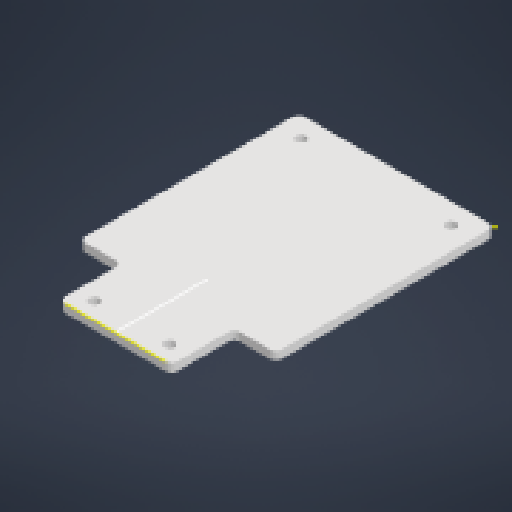
# Autodesk Inventor part: 1.5_base_2
Saved by Autodesk Inventor 2025 (Build 290162010, 162A)
## iProperties
Created: 2024-05-22
Part Number: 1.5_base_2
Material: Generic
Document SubType Name: Modeling
Designer: Garfieldcmix
Density: 1 g/cm^3
Appearance: Default
Author: Garfieldcmix
Autodesk Inventor part; units mm, degrees
ref_plane "YZ Plane" through (0, 0, 0) normal (1, 0, 0) x (0, 1, 0)
ref_plane "XZ Plane" through (0, 0, 0) normal (0, 1, 0) x (-1, 0, 0)
ref_plane "XY Plane" through (0, 0, 0) normal (0, 0, 1) x (1, 0, 0)
derived "Car_Plan.ipt"
sketch "Car_Sketch" plane through (0, 0, 0) normal (0, 1, 0) x (-1, 0, 0)
  line L0 (0, 0) -> (94, 0)
  line L1 (0, 0) -> (0, 105)
  line L2 (94, 0) -> (94, 105)
  line L3 (0, 105) -> (20, 105)
  line L4 (20, 105) -> (20, 190)
  line L5 (20, 190) -> (74, 190)
  line L6 (74, 190) -> (74, 105)
  line L7 (74, 105) -> (94, 105)
  line L8 (-5, 68) -> (-5, 0)
  line L9 (-5, 0) -> (-32, 0)
  line L10 (-32, 0) -> (-32, 68)
  line L11 (-32, 68) -> (-5, 68)
  line L12 (47, 190) -> (47, 0) construction
  line L13 (126, 68) -> (99, 68)
  line L14 (99, 68) -> (99, 0)
  line L15 (126, 0) -> (126, 68)
  line L16 (99, 0) -> (126, 0)
  line L17 (-5, 34) -> (99, 34) construction
  line L18 (0, 95) -> (94, 95) construction
  line L19 (-5, 190) -> (-32, 190)
  line L20 (-32, 122) -> (-5, 122)
  line L21 (-32, 190) -> (-32, 122)
  line L22 (-5, 122) -> (-5, 190)
  line L23 (-5, 156) -> (99, 156) construction
  line L24 (126, 122) -> (99, 122)
  line L25 (126, 190) -> (126, 122)
  line L26 (99, 190) -> (126, 190)
  line L27 (99, 122) -> (99, 190)
  line L28 (0, 156) -> (47, 34) construction
  line L29 (94, 156) -> (47, 34) construction
  line L30 (0, 156) -> (-174.2341, 34) construction
  line L31 (-5, 34) -> (-174.2341, 34) construction
  line L32 (8.9873, 132.6713) -> (47, 141.55) construction
  line L33 (85.0127, 132.6713) -> (47, 141.55) construction
sketch "Base" plane through (0, 0, 0) normal (0, 1, 0) x (-1, 0, 0)
  line L0 (0, 0) -> (0, 105) projected
  line L1 (0, 105) -> (20, 105) projected
  line L2 (20, 105) -> (20, 190) projected
  line L3 (74, 190) -> (74, 105) projected
  line L4 (74, 105) -> (94, 105) projected
  line L5 (94, 0) -> (94, 105) projected
  line L6 (0, 0) -> (94, 0) projected
  line L7 (74, 135) -> (20, 135)
  circle A0 centre (29, 127) radius 2.4
  circle A1 centre (65, 127) radius 2.4
  circle A2 centre (11.1, 10) radius 2.4
  circle A3 centre (82.9, 10) radius 2.4
  dimension "d76" = 30
  dimension "d77" = 4.8
  dimension "d78" = 4.8
  dimension "d79" = 9
  dimension "d80" = 22
  dimension "d81" = 22
  dimension "d82" = 9
  dimension "d83" = 4.8
  dimension "d84" = 4.8
  dimension "d85" = 10
  dimension "d86" = 11.1
  dimension "d87" = 10
  dimension "d88" = 11.1
  constraints: 4 centre point, 2 end point, 2 point on line, 1 perpendicular
  measures "d76" distance between parallel lines of L1 L7
  measures "d77" diameter of A0
  measures "d78" diameter of A1
  measures "d79" distance from line of L2 A0.centre
  measures "d80" distance from line of L1 A0.centre
  measures "d81" distance from line of A1.centre L4
  measures "d82" distance from line of L3 A1.centre
  measures "d83" diameter of A2
  measures "d84" diameter of A3
  measures "d85" distance from line of L6 A2.centre
  measures "d86" distance from line of L0 A2.centre
  measures "d87" distance from line of L6 A3.centre
  measures "d88" distance from line of L5 A3.centre
extrude "Extrusion1" add sketch "Base" along normal blind 4
fillet "Fillet2" radius 3 8 edges at (-20, 2, 105) (0, 2, 105) (0, 2, 0) (-94, 2, 0) (-94, 2, 105) (-74, 2, 105) (-74, 2, 135) (-20, 2, 135)
sketch "Sketch19" plane through (0, 4, 0) normal (0, 1, 0) x (1, 0, 0)
  line L0 (0, -102) -> (0, -3) projected
  line L1 (-17, -105) -> (-3, -105) projected
  line L2 (-94, -3) -> (-94, -102) projected
  line L3 (-91, -105) -> (-77, -105) projected
  line L4 (0, -100.2906) -> (-4.5, -100.2906)
  line L5 (-4.5, -100.2906) -> (-89.5, -100.2906)
  line L6 (-89.5, -100.2906) -> (-89.5, -44.2906)
  line L7 (-89.5, -44.2906) -> (-4.5, -44.2906)
  line L8 (-4.5, -44.2906) -> (-4.5, -100.2906)
  line L9 (-4.5, -100.2906) -> (-8, -100.2906)
  line L10 (-4.5, -96.7906) -> (-4.5, -100.2906)
  circle A0 centre (-28, -96.7906) radius 1.35
  line L11 (-28, -96.7906) -> (-24.5, -96.7906)
  line L12 (-24.5, -96.7906) -> (-24.5, -100.2906)
  line L13 (-24.5, -100.2906) -> (-28, -100.2906)
  line L14 (-28, -100.2906) -> (-28, -96.7906)
  line L15 (-24.5, -100.2906) -> (-89.5, -100.2906)
  line L16 (-89.5, -100.2906) -> (-89.5, -44.2906)
  line L17 (-89.5, -44.2906) -> (-24.5, -44.2906)
  line L18 (-24.5, -44.2906) -> (-24.5, -100.2906)
  line L19 (-57, -100.2906) -> (-57, -87.065)
  line L20 (-24.5, -72.2906) -> (-39.3063, -72.2906)
  circle A1 centre (-86, -96.7906) radius 1.35
  circle A2 centre (-28, -47.7906) radius 1.35
  circle A3 centre (-86, -47.7906) radius 1.35
  point P0 (0, 0)
  dimension "d196" = 4.5
  dimension "d197" = 85
  dimension "d198" = 56
  dimension "d199" = 4.7095
  dimension "d202" = 2.7
  dimension "d203" = 3.5
  dimension "d204" = 23.5
  dimension "d205" = 3.5
  constraints: 34 end point, 6 horizontal, 6 parallel, 4 centre point, 3 perpendicular, 3 symmetric about line, 2 midpoint, 2 point on line, 1 vertical, 3 other
  measures "d196" distance of L4.start L4.end
  measures "d197" distance of L6.end L7.end
  measures "d198" distance of L5.end L6.end
  measures "d199" distance between parallel lines of L1 L4
  measures "d202" diameter of A0
  measures "d203" distance from line of L5 L11.start
  measures "d204" distance from line of L8 L11.start
  measures "d205" distance of L12.end L13.end
extrude "Extrusion12" cut sketch "Sketch19" against normal through all contours L14 L11 A0 | A0 L11 L14 | A1 | A2 | A3
sketch "Sketch20" plane through (0, 4, 0) normal (0, 1, 0) x (1, 0, 0)
  line L0 (0, -102) -> (0, -3) projected
  line L1 (0, -4.0657) -> (-25.4, -4.0657)
  line L2 (-3, 0) -> (-91, 0) projected
  line L3 (-25.4, -4.0657) -> (-68.58, -4.0657)
  line L4 (-68.58, -4.0657) -> (-68.58, -39.6257)
  line L5 (-68.58, -39.6257) -> (-25.4, -39.6257)
  line L6 (-25.4, -39.6257) -> (-25.4, -4.0657)
  line L7 (-25.4, -39.6257) -> (-27.94, -39.6257)
  line L8 (-27.94, -39.6257) -> (-27.94, -37.0857)
  line L9 (-27.94, -37.0857) -> (-25.4, -37.0857)
  line L10 (-25.4, -37.0857) -> (-25.4, -39.6257)
  circle A0 centre (-27.94, -37.0857) radius 1.5
  line L11 (-46.99, -39.6257) -> (-46.99, -31.1467)
  line L12 (-25.4, -21.8457) -> (-34.7805, -21.8457)
  circle A1 centre (-66.04, -37.0857) radius 1.5
  circle A2 centre (-27.94, -6.6057) radius 1.5
  circle A3 centre (-66.04, -6.6057) radius 1.5
  point P0 (0, 0)
  dimension "d208" = 25.4
  dimension "d209" = 4.0657
  dimension "d210" = 43.18
  dimension "d211" = 35.56
  dimension "d212" = 2.54
  dimension "d213" = 2.54
  dimension "d214" = 3
  constraints: 22 end point, 4 centre point, 4 parallel, 3 horizontal, 3 perpendicular, 3 symmetric about line, 2 midpoint, 1 coincident, 1 point on line, 1 vertical, 3 other
  measures "d208" distance of L1.start L1.end
  measures "d209" distance between parallel lines of L2 L1
  measures "d210" distance of L5.end L4.end
  measures "d211" distance of L4.end L3.end
  measures "d212" distance of L8.end L9.end
  measures "d213" distance of L7.end L8.end
  measures "d214" diameter of A0
extrude "Extrusion13" cut sketch "Sketch20" against normal through all contours A0 L8 L9 | L9 L8 A0 | A1 | A2 | A3
body "Solid1"
